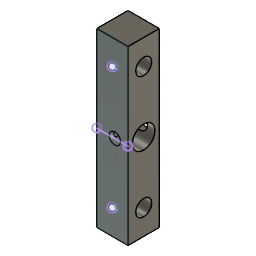
ElecMagBar (Autodesk Fusion 360 design; units mm, degrees)
part number: 2025-12-16-09-55-40-049
Autodesk Fusion 360 part; units mm, degrees
note: some values were not read from the file. Set by a fixed rule: which face or edge a step refers to.
box "BoxPrimitive1" add length 12.5 width 12.5 height 68.75 placed x (0, 1, 0) y (-1, 0, 0) z (0, 0, 1) at (12.5, 0, 0)
sketch "Sketch2" plane through (12.5, 0, 0) normal (1, 0, 0) x (0, 1, 0)
  line L0 (0, 68.75) -> (0, 0)
  line L1 (0, 0) -> (12.5, 0)
  line L2 (12.5, 0) -> (12.5, 68.75)
  line L3 (12.5, 68.75) -> (0, 68.75)
  line L4 (0, 34.375) -> (12.5, 34.375)
  line L5 (6.25, 0) -> (6.25, 10)
  point P0 (6.25, 34.375)
  point P1 (6.25, 58.75)
  dimension "d37" = 10
  constraint midpoint L0 L4.start
  constraint midpoint L2 L4.end
  constraint midpoint L1 L5.start
  constraint perpendicular L1 L5
  constraint symmetric L4 L5.end P1
  measures "d37" distance of L5.start L5.end
hole "Hole1" at (12.5, 6.25, 34.375) at (12.5, 6.25, 10) at (12.5, 6.25, 58.75) direction (-1, 0, 0) diameter 6.35 depth 11 tip angle 180
sketch "Sketch3" plane through (0, 12.5, 0) normal (0, 1, 0) x (-1, 0, 0)
  line L0 (-12.5, 68.75) -> (-12.5, 0)
  line L1 (-12.5, 0) -> (0, 0)
  line L2 (0, 0) -> (0, 68.75)
  line L3 (0, 68.75) -> (-12.5, 68.75)
  circle A0 centre (-7.25, 34.375) radius 2
  dimension "d12" = 4
  measures "d12" diameter of A0
extrude "Extrude1" cut sketch "Sketch3" against normal blind 13 contours A0
extrude "Extrude2" cut 1 faces at (1.5, 5.5302, 10.7758) along direction (-1, 0, 0) blind 32
extrude "Extrude3" cut 1 faces at (1.5, 7.1817, 57.1788) along direction (-1, 0, 0) blind 72
cylinder "CylinderPrimitive1" cut diameter 4 height -5 placed x (0, 0, -1) y (0, 1, 0) z (1, 0, 0) at (1.5, 6.25, 34.375)
extrude "Extrude4" add 1 faces at (1.5, 6.5071, 31.6109) along direction (1, 0, 0) blind 1
sketch "Sketch5" plane through (0, 12.5, 0) normal (0, 1, 0) x (-1, 0, 0)
  circle A0 centre (-7.25, 34.375) radius 2
  line L0 (-12.5, 68.75) -> (-12.5, 0)
  line L1 (-12.5, 0) -> (0, 0)
  line L2 (0, 0) -> (0, 68.75)
  line L3 (0, 68.75) -> (-12.5, 68.75)
  line L4 (-12.5, 34.375) -> (0, 34.375)
  line L5 (-6.25, 0) -> (-6.25, 10)
  circle A1 centre (-6.25, 10) radius 1
  circle A2 centre (-6.25, 58.75) radius 1
  dimension "d43" = 10
  dimension "d44" = 2
  constraint midpoint L0 L4.start
  constraint midpoint L2 L4.end
  constraint midpoint L1 L5.start
  constraint perpendicular L1 L5
  constraint coincident L5.end A1.centre
  constraint symmetric L4 A1 A2
  measures "d43" distance of L5.start L5.end
  measures "d44" diameter of A1
hole "Hole2" at (6.25, 12.5, 10) at (6.25, 12.5, 58.75) direction (0, -1, 0) diameter 2.5 depth 17 tip angle 180
hole "Hole3" at (12.5, 6.25, 34.375) direction (-1, 0, 0) diameter 9.5 depth 10 tip angle 180
move_face "OffsetFaces3" offset -0.25 2 faces at (2.1667, 6.0509, 32.3849) (1, 6.0509, 32.3849)
sketch "Sketch6" plane through (0, 0, 0) normal (0, -1, 0) x (1, 0, 0)
  circle A0 centre (7.25, 34.375) radius 2
  line L0 (0, 68.75) -> (0, 0)
  line L1 (0, 0) -> (12.5, 0)
  line L2 (12.5, 0) -> (12.5, 68.75)
  line L3 (12.5, 68.75) -> (0, 68.75)
  line L4 (6.25, 10.025) -> (7.9, 10.025)
  line L5 (7.9, 10.025) -> (7.075, 9.0859)
  line L6 (7.075, 9.0859) -> (7.9, 10.025)
  line L7 (7.9, 10.025) -> (7.075, 10.9641)
  line L8 (7.075, 10.9641) -> (7.075, 9.0859)
  line L9 (12.5, 34.375) -> (0, 34.375)
  circle A1 centre (6.25, 10) radius 1.25
  circle A2 centre (6.25, 58.75) radius 1.25
  line L10 (7.075, 57.7859) -> (7.075, 59.6641)
  line L11 (7.9, 58.725) -> (7.075, 59.6641)
  line L12 (6.25, 58.725) -> (7.9, 58.725)
  line L13 (7.9, 58.725) -> (7.075, 57.7859)
  constraint horizontal L4
  constraint perpendicular L4 L8
  constraint symmetric L4.start L9 L12.start
  constraint symmetric L4.end L9 L11.start
  constraint symmetric L5.end L9 L10.end
  constraint symmetric L7.end L9 L10.start
extrude "Extrude5" cut sketch "Sketch6" against normal blind 13 contours L4 L7 L8 A1 | L4 L5 L6 A1 | A2 L11 L12 | A2 L10 L12 L13
move_face "OffsetFaces4" offset -0.25 2 faces at (7.2555, 11.8528, 36.375) (7.2555, 0.6472, 36.375)
move_face "OffsetFaces5" offset 0.25 1 faces at (7.3989, 10.1345, 31.6413)
